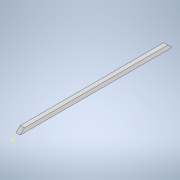
# Autodesk Inventor part: TopTop
Saved by Autodesk Inventor 2020.1 (Build 241239000, 239)
## iProperties
Created: 2019-12-20
Part Number: TopTop
Material: Generic
Document SubType Name: Modeling
Designer: super
Density: 1 g/cm^3
Appearance: Default
Author: super
Autodesk Inventor part; units mm, degrees
ref_plane "YZ Plane" through (0, 0, 0) normal (1, 0, 0) x (0, 1, 0)
ref_plane "XZ Plane" through (0, 0, 0) normal (0, 1, 0) x (-1, 0, 0)
ref_plane "XY Plane" through (0, 0, 0) normal (0, 0, 1) x (1, 0, 0)
sketch "Sketch1" plane through (0, 0, 0) normal (0, 1, 0) x (-1, 0, 0)
  line L0 (0, 0) -> (-6.35, 0)
  line L1 (-6.35, 0) -> (-6.35, -244)
  line L2 (-6.35, -244) -> (0, -244)
  line L3 (0, -244) -> (0, 0)
  dimension "d0" = 6.35
  dimension "d1" = 244
  constraints: 8 end point, 2 parallel, 1 horizontal, 1 perpendicular
  measures "d0" distance of L2.end L1.end
  measures "d1" distance of L1.end L0.end
extrude "Extrusion1" add sketch "Sketch1" along normal blind 6.35
sketch "Sketch2" plane through (6.35, 0, 0) normal (1, 0, 0) x (0, 0, -1)
  line L0 (0, 0) -> (244, 0) projected
  line L1 (0, 0) -> (6.35, 6.35)
  line L2 (0, 6.35) -> (244, 6.35) projected
  line L3 (0, 0) -> (8.9803, 0) construction
  line L4 (6.35, 6.35) -> (0, 6.35)
  line L5 (0, 6.35) -> (0, 0)
  dimension "d4" = 45
  constraints: 8 end point, 2 point on line, 1 collinear, 1 equal length, 1 horizontal, 1 perpendicular
  measures "d4" angle of L3 L1
extrude "Extrusion2" cut sketch "Sketch2" against normal blind 10
sketch "Sketch3" plane through (6.35, 0, -244) normal (1, 0, 0) x (0, 0, -1)
  line L0 (0, 0) -> (-6.35, 6.35)
  line L1 (0, 6.35) -> (-237.65, 6.35) projected
  line L2 (0, 0) -> (8.9803, 0) construction
  line L3 (-6.35, 6.35) -> (0, 6.35)
  line L4 (0, 6.35) -> (0, 0)
  point P0 (-244, 0)
  dimension "d7" = 135
  constraints: 8 end point, 1 collinear, 1 equal length, 1 horizontal, 1 perpendicular, 1 point on line
  measures "d7" angle of L2 L0
extrude "Extrusion3" cut sketch "Sketch3" against normal blind 10
sketch "Sketch4" plane through (6.35, 0, 0) normal (1, 0, 0) x (0, 0, -1)
  line L0 (0, 0) -> (6.35, 6.35) projected
  line L1 (244, 0) -> (0, 0) projected
  line L2 (6.35, 0) -> (12.4246, 0)
  line L3 (237.65, 6.35) -> (6.35, 6.35) projected
  line L4 (12.4246, 6.35) -> (12.4246, 0)
  line L5 (12.4246, 6.35) -> (6.35, 6.35)
  line L6 (0, 0) -> (6.35, 0)
  line L7 (0, 0) -> (6.35, 6.35)
  dimension "d11" = 6.35
  constraints: 10 end point, 3 collinear, 3 point on line, 1 perpendicular
  measures "d11" distance of L0.end L2.start
extrude "Extrusion4" cut sketch "Sketch4" against normal blind 10
sketch "Sketch5" plane through (6.35, 0, -12.4246) normal (1, 0, 0) x (0, 0, -1)
  point P0 (-12.4246, 0)
sketch "Sketch6" plane through (6.35, 0, -12.4246) normal (1, 0, 0) x (0, 0, -1)
  line L0 (0, 6.35) -> (0, 0) projected
  line L1 (0, 0) -> (6.35, 6.35)
  line L2 (225.2254, 6.35) -> (0, 6.35) projected
  line L3 (0, 0) -> (8.9803, 0) construction
  line L4 (6.35, 6.35) -> (0, 6.35)
  line L5 (231.5754, 0) -> (0, 0) projected
  line L6 (0, 6.35) -> (0, 0)
  point P0 (-12.4246, 0)
  dimension "d14" = 45
  constraints: 8 end point, 1 collinear, 1 equal length, 1 horizontal, 1 perpendicular, 1 point on line
  measures "d14" angle of L3 L1
extrude "Extrusion5" cut sketch "Sketch6" against normal blind 10
body "Solid1"
